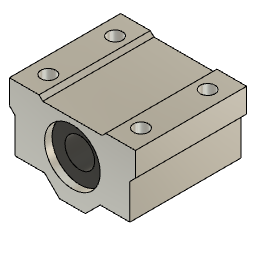
Pillow Block 8mm (Autodesk Fusion 360 design; units mm, degrees)
Autodesk Fusion 360 part; units mm, degrees
sketch "Front" plane through (0, 0, 0) normal (0, 1, 0) x (1, 0, 0)
  circle A0 centre (0, 0) radius 4
  circle A1 centre (0, 0) radius 7.5
  line L0 (0, 0) -> (0, -15) construction
  line L1 (-18.6476, -9) -> (-14.6519, -9) construction
  line L2 (-14.6519, -9) -> (18.8366, -9) construction
  line L3 (-17, -10) -> (18.8681, -10) construction
  line L4 (-15, 7.5) -> (15, 7.5) construction
  line L5 (-15, 11.5) -> (15, 11.5) construction
  line L6 (0, -9) -> (8, -9)
  line L7 (8, -9) -> (9, -10)
  line L8 (9, -10) -> (17, -10)
  line L9 (17, -10) -> (17, -3.5)
  line L10 (17, -3.5) -> (15.5, -2)
  line L11 (15.5, -2) -> (15.5, 7.5)
  line L12 (7.5, 7.5) -> (3.5, 11.5)
  line L13 (-3.5, 11.5) -> (-7.5, 7.5)
  line L14 (-15.5, 7.5) -> (-15.5, -2)
  line L15 (-15.5, -2) -> (-17, -3.5)
  line L16 (-17, -3.5) -> (-17, -10)
  line L17 (-9, -10) -> (-8, -9)
  line L18 (0, -9) -> (-8, -9)
  line L19 (-17, -10) -> (-9, -10)
  line L20 (-7.5, 7.5) -> (-15.5, 7.5)
  line L21 (15.5, 7.5) -> (7.5, 7.5)
  line L22 (3.5, 11.5) -> (-3.5, 11.5)
  dimension "d1" = 8
  dimension "d2" = 15
  dimension "d5" = 9
  dimension "d6" = 10
  dimension "d7" = 7.5
  dimension "d8" = 11.5
  dimension "d9" = 15.5
  dimension "d10" = 15.5
  dimension "d11" = 1.5
  dimension "d12" = 1.5
  dimension "d13" = 1.5
  dimension "d14" = 1.5
  dimension "d15" = 16
  dimension "d16" = 4
  dimension "d17" = 4
  dimension "d18" = 6.5
  dimension "d19" = 9.5
  dimension "d20" = 8
  dimension "d21" = 8
  dimension "d22" = 1
  constraint coincident A0.centre A1.centre
  constraint vertical L0
  constraint perpendicular L0 L2
  constraint perpendicular L0 L3
  constraint horizontal L4
  constraint horizontal L5
  constraint coincident L0 L6.start
  constraint coincident L2 L6.start
  constraint coincident L2 L6.end
  constraint coincident L3 L7.end
  constraint coincident L3 L8.end
  constraint parallel L7 L10
  constraint coincident L4 L12.start
  constraint coincident L5 L12.end
  constraint coincident L5 L13.start
  constraint coincident L3 L17.start
  constraint coincident L2 L17.end
  constraint parallel L15 L17
  constraint perpendicular L14 L20
  constraint equal L8 L19
  constraint equal L9 L16
  constraint equal L11 L14
  constraint equal L20 L21
  constraint equal L12 L13
  constraint perpendicular L16 L19
  constraint parallel L9 L11
  constraint parallel L14 L16
  constraint perpendicular L10 L15
  constraint horizontal L21
  measures "d1" diameter of A0
  measures "d2" diameter of A1
  measures "d5" distance of A0.centre L2
  measures "d6" distance of A0.centre L3
  measures "d7" distance of A0.centre L4
  measures "d8" distance of A0.centre L5
  measures "d9" distance of L0 L11
  measures "d10" distance of L0 L14
  measures "d11" distance of L9 L11
  measures "d12" vertical distance of L9.end L10.end
  measures "d13" distance of L14 L16
  measures "d14" vertical distance of L14.end L15.end
  measures "d15" distance of L6.end L17.end
  measures "d16" horizontal distance of L12.start L12.end
  measures "d17" vertical distance of L12.start L12.end
  measures "d18" distance of L3 L15.end
  measures "d19" distance of L14.start L14.end
  measures "d20" distance of L3.start L17.start
  measures "d21" distance of L13.end L14.start
  measures "d22" distance of L3 L6
extrude "Extrude1" add sketch "Front" along normal blind 30 contours L6 L7 L8 L9 L10 L11 L12 L13 L14 L15 L16 L17 L18 L19 L20 L21 L22
extrude "Extrude2" add sketch "Front" along normal blind 28 contours A1
extrude "Extrude3" cut sketch "Front" along normal blind 2 contours A1
sketch "Top" plane through (0, 0, 10) normal (0, 0, 1) x (-1, 0, 0)
  line L0 (17, 0) -> (9, 0)
  line L1 (9, 0) -> (9, -30)
  line L2 (9, -30) -> (17, -30)
  line L3 (17, -30) -> (17, 0)
  line L4 (17, -30) -> (-17, 0) construction
  line L5 (-17, -30) -> (17, 0) construction
  line L6 (-12.5, -24) -> (12.5, -24) construction
  line L7 (12.5, -24) -> (12.5, -6) construction
  line L8 (12.5, -6) -> (-12.5, -6) construction
  line L9 (-12.5, -6) -> (-12.5, -24) construction
  line L10 (-12.5, -24) -> (12.5, -6) construction
  line L11 (12.5, -24) -> (-12.5, -6) construction
  circle A0 centre (12.5, -24) radius 2
  circle A1 centre (-12.5, -24) radius 2
  circle A2 centre (-12.5, -6) radius 2
  circle A3 centre (12.5, -6) radius 2
  point P0 (0, -15)
  dimension "d29" = 25
  dimension "d30" = 18
  dimension "d31" = 4
  dimension "d32" = 4
  dimension "d33" = 4
  dimension "d34" = 4
  constraint coincident L2.end L3.start
  constraint coincident L0.start L3.end
  constraint perpendicular L6 L7
  constraint parallel L6 L8
  constraint parallel L7 L9
  constraint horizontal L6
  constraint coincident L10 P0
  constraint coincident L11 P0
  constraint midpoint L5 P0
  constraint coincident L6.end L7.start
  constraint coincident L6.start L9.end
  constraint coincident L8.end L9.start
  constraint coincident L7.end L8.start
  measures "d29" distance of L7.end L8.end
  measures "d30" distance of L6.end L7.end
  measures "d31" diameter of A0
  measures "d32" diameter of A1
  measures "d33" diameter of A2
  measures "d34" diameter of A3
extrude "Extrude4" cut sketch "Top" against normal blind 27 contours A0 | A1 | A2 | A3
named bodies: "Pillow block"
